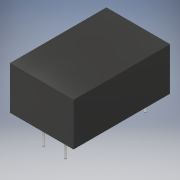
# Autodesk Inventor part: IRM-02-5
Saved by Autodesk Inventor 2018 (Build 220112000, 112)
## iProperties
Created: 2018-03-01
Part Number: IRM-02-5
Material: Generic
Document SubType Name: Modeling
Designer: brutu
Density: 1 g/cm^3
Appearance: Default
Author: brutu
Autodesk Inventor part; units mm, degrees
ref_plane "YZ Plane" through (0, 0, 0) normal (1, 0, 0) x (0, 1, 0)
ref_plane "XZ Plane" through (0, 0, 0) normal (0, 1, 0) x (-1, 0, 0)
ref_plane "XY Plane" through (0, 0, 0) normal (0, 0, 1) x (1, 0, 0)
sketch "Sketch1" plane through (0, 0, 0) normal (0, 1, 0) x (-1, 0, 0)
  line L0 (11.1, 16.85) -> (-11.1, 16.85)
  line L1 (-11.1, 16.85) -> (-11.1, -16.85)
  line L2 (-11.1, -16.85) -> (11.1, -16.85)
  line L3 (11.1, -16.85) -> (11.1, 16.85)
  point P0 (0, 0)
  dimension "d0" = 33.7
  dimension "d1" = 22.2
  dimension "d2" = 16.85
  dimension "d3" = 11.1
  constraints: 8 end point, 2 parallel, 1 horizontal, 1 perpendicular
  measures "d0" distance of L2.end L0.start
  measures "d1" distance of L0.start L0.end
  measures "d2" distance from line of L0 point (0, 0)
  measures "d3" distance from line of L1 point (0, 0)
extrude "Extrusion1" add sketch "Sketch1" along normal blind 15
sketch "Sketch2" plane through (0, 0, 0) normal (0, -1, 0) x (1, 0, 0)
  circle A0 centre (5.3802, 14) radius 0.35
  circle A1 centre (-2.2198, 14) radius 0.35
  circle A2 centre (5.3802, -14) radius 0.35
  circle A3 centre (-9.8198, -14) radius 0.35
  line L0 (-11.1, 16.85) -> (11.1, 16.85) projected
  line L1 (-11.1, -16.85) -> (-11.1, 16.85) projected
  line L2 (11.1, -16.85) -> (-11.1, -16.85) projected
  line L3 (11.1, 16.85) -> (11.1, -16.85) projected
  point P0 (0, 0)
  dimension "d6" = 0.7
  dimension "d7" = 0.7
  dimension "d8" = 0.7
  dimension "d9" = 0.7
  dimension "d10" = 7.6
  dimension "d11" = 15.2
  dimension "d12" = 28
  dimension "d14" = 2.85
  constraints: 4 centre point, 2 horizontal alignment, 1 vertical alignment
  measures "d6" diameter of A0
  measures "d7" diameter of A2
  measures "d8" diameter of A1
  measures "d9" diameter of A3
  measures "d10" distance of A1.centre A0.centre
  measures "d11" distance of A3.centre A2.centre
  measures "d12" distance of A2.centre A0.centre
  measures "d14" distance from line of L2 A2.centre
extrude "Extrusion2" add sketch "Sketch2" along normal blind 7 contours A0 | A1 | A2 | A3
equation "\"d2\" = 0.5 * d0"
equation "\"d3\" = 0.5 * d1"
equation "\"d7\" = d6"
equation "\"d8\" = d6"
equation "\"d9\" = d6"
body "Solid1"
